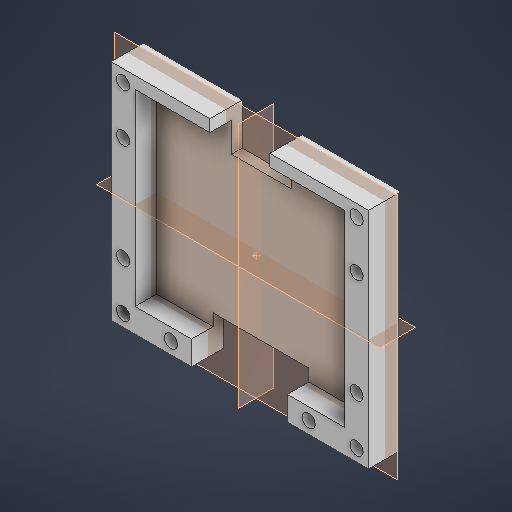
# Autodesk Inventor part: Checkpoint10.2_BackCover
Saved by Autodesk Inventor 2026.1 (Build 301233020, 233B)
## iProperties
Created: 2025-10-03
Part Number: Checkpoint10.2_BackCover
Material: Generic
Document SubType Name: Modeling
Designer: ghimirea
Density: 1 g/cm^3
Appearance: Default
Author: ghimirea
Autodesk Inventor part; units mm, degrees
sketch "Sketch1" plane through (0, 0, 0) normal (0, 0, 1) x (1, 0, 0)
  line L0 (-10.75, -9.35) -> (10.75, -9.35)
  line L1 (10.75, -9.35) -> (10.75, 9.35)
  line L2 (10.75, 9.35) -> (-10.75, 9.35)
  line L3 (-10.75, 9.35) -> (-10.75, -9.35)
  line L4 (-10.75, -9.35) -> (10.75, 9.35) construction
  line L5 (10.75, -9.35) -> (-10.75, 9.35) construction
  point P0 (0, 0)
  dimension "d0" = 21.5
  dimension "d1" = 18.7
  constraints: 12 end point, 2 midpoint, 2 parallel, 1 horizontal, 1 perpendicular
  measures "d0" distance of L0.start L0.end
  measures "d1" distance of L1.end L0.end
extrude "Extrusion1" add sketch "Sketch1" along normal mid plane 2.7
sketch "Sketch3" plane through (0, 0, 1.35) normal (0, 0, 1) x (1, 0, 0)
  line L0 (-8.75, -7.35) -> (8.75, -7.35)
  line L1 (8.75, -7.35) -> (8.75, 8.35)
  line L2 (8.75, 8.35) -> (-8.75, 8.35)
  line L3 (-8.75, 8.35) -> (-8.75, -7.35)
  line L4 (-8.75, -7.35) -> (8.75, 8.35) construction
  line L5 (8.75, -7.35) -> (-8.75, 8.35) construction
  line L6 (-10.75, -9.35) -> (10.75, -9.35)
  point P0 (0, 0.5)
  dimension "d8" = 17.5
  dimension "d47" = 2
  dimension "d61" = 15.7
  constraints: 14 end point, 2 midpoint
  measures "d8" distance of L0.start L0.end
  measures "d47" distance between parallel lines of L6 L0
  measures "d61" distance between parallel lines of L0 L2
extrude "Extrusion3" cut sketch "Sketch3" against normal blind 1.8
sketch "Sketch4" plane through (0, 0, 1.35) normal (0, 0, 1) x (1, 0, 0)
  line L0 (2.5, 5.884) -> (-2.5, 5.884)
  line L1 (-2.5, 5.884) -> (-2.5, 12.884)
  line L2 (-2.5, 12.884) -> (2.5, 12.884)
  line L3 (2.5, 12.884) -> (2.5, 5.884)
  line L4 (2.5, 5.884) -> (-2.5, 12.884) construction
  line L5 (-2.5, 5.884) -> (2.5, 12.884) construction
  point P0 (0, 0)
  point P1 (0, 9.384)
  dimension "d12" = 5
  dimension "d15" = 7
  constraints: 12 end point, 2 midpoint, 2 parallel, 1 horizontal, 1 perpendicular
  measures "d12" distance of L0.start L0.end
  measures "d15" distance between parallel lines of L0 L2
extrude "Extrusion4" cut sketch "Sketch4" against normal blind 3
sketch "Sketch7" plane through (-10.75, 0.5, 6.442) normal (1, 0, 0) x (0, -1, 0)
  line L0 (3.5, 6.442) -> (-2.5, 6.442)
  line L1 (-2.5, 6.442) -> (-2.5, 9.442)
  line L2 (-2.5, 9.442) -> (3.5, 9.442)
  line L3 (3.5, 9.442) -> (3.5, 6.442)
  line L4 (3.5, 6.442) -> (-2.5, 9.442) construction
  line L5 (-2.5, 6.442) -> (3.5, 9.442) construction
  line L6 (0.5, -1.8884) -> (0.5, 11.3304) projected
  line L7 (-8.85, 7.792) -> (-8.85, 5.092) projected
  point P0 (0, 0)
  point P1 (0.5, 7.942)
  point P2 (0.5, 7.942)
  point P3 (0.5, -1.8884)
  point P4 (0.5, 11.3304)
  point P5 (-8.85, 6.442)
  dimension "d24" = 6
  dimension "d23" = 3
  constraints: 12 end point, 4 midpoint, 2 parallel, 1 horizontal, 1 perpendicular, 1 point on line, 2 other
  measures "d24" distance of L0.start L0.end
  measures "d23" distance between parallel lines of L0 L2
extrude "Extrusion7" [suppressed]
fillet "Fillet1" [suppressed]
fillet "Fillet2" [suppressed]
fillet "Fillet3" [suppressed]
fillet "Fillet4" [suppressed]
fillet "Fillet5" [suppressed]
fillet "Fillet6" radius 0.2 1 edges at (10.75, 0, -1.35)
fillet "Fillet7" [suppressed]
fillet "Fillet8" [suppressed]
fillet "Fillet9" [suppressed]
fillet "Fillet10" [suppressed]
fillet "Fillet11" [suppressed]
mirror "Mirror2" [suppressed]
sketch "InsertPoles_Sketch" plane through (0, 0, 1.35) normal (0, 0, 1) x (1, 0, 0)
  circle A0 centre (-9.75, -8.35) radius 0.55
  line L0 (-10.75, 9.35) -> (-10.75, -9.35) projected
  line L1 (-10.75, -9.35) -> (10.75, -9.35) projected
  circle A1 centre (-9.75, -4.35) radius 0.55
  circle A2 centre (-9.75, 4.35) radius 0.55
  circle A3 centre (-9.75, 8.35) radius 0.55
  circle A4 centre (-5.75, -8.35) radius 0.55
  line L2 (-2.5, 9.35) -> (-10.75, 9.35) projected
  point P0 (0, 0)
  point P1 (-8.75, 9.35)
  dimension "d39" = 1.1
  dimension "d40" = 1
  dimension "d41" = 1
  dimension "d42" = 1.1
  dimension "d43" = 1.1
  dimension "d44" = 1.1
  dimension "d45" = 1.1
  dimension "d48" = 4
  dimension "d49" = 1
  dimension "d50" = 1
  dimension "d51" = 4
  dimension "d52" = 4
  constraints: 5 centre point
  measures "d39" diameter of A0
  measures "d40" distance from line of A0.centre L0
  measures "d41" distance from line of L1 A0.centre
  measures "d42" diameter of A1
  measures "d43" diameter of A2
  measures "d44" diameter of A3
  measures "d45" diameter of A4
  measures "d48" distance of A0.centre A1.centre
  measures "d49" distance from line of L2 A3.centre
  measures "d50" distance from line of L0 A3.centre
  measures "d51" distance of A2.centre A3.centre
  measures "d52" distance of A4.centre A0.centre
extrude "InsertPoles_Extrude" cut sketch "InsertPoles_Sketch" against normal blind 3
mirror "MirrorInsertPoles" about plane through (0, 0, 0) normal (1, 0, 0) of "InsertPoles_Extrude"
sketch "RibbonCableCutout_Sketch" plane through (0, 0, 1.35) normal (0, 0, 1) x (1, 0, 0)
  line L0 (3, -7.0087) -> (-3, -7.0087)
  line L1 (-3, -7.0087) -> (-3, -9.0087)
  line L2 (-3, -9.0087) -> (3, -9.0087)
  line L3 (3, -9.0087) -> (3, -7.0087)
  line L4 (3, -7.0087) -> (-3, -9.0087) construction
  line L5 (-3, -7.0087) -> (3, -9.0087) construction
  line L6 (0, 13.09) -> (0, -13.09) projected
  point P0 (0, 0)
  point P1 (0, -8.0087)
  point P2 (0, -8.0087)
  dimension "d56" = 6
  dimension "d57" = 2
  constraints: 12 end point, 3 midpoint, 2 parallel, 1 horizontal, 1 perpendicular, 1 point on line
  measures "d56" distance of L0.start L0.end
  measures "d57" distance of L1.end L0.end
extrude "RibbonCableCutout_Extrude" [suppressed]
fillet "Fillet12" [suppressed]
sketch "Sketch11" plane through (-0.0016, -9.35, -6.4418) normal (0, -1, 0) x (1, 0, 0)
  line L0 (3.9693, 3.0494) -> (-4.0307, 3.0494)
  line L1 (-4.0307, 3.0494) -> (-4.0307, 10.0494)
  line L2 (-4.0307, 10.0494) -> (3.9693, 10.0494)
  line L3 (3.9693, 10.0494) -> (3.9693, 3.0494)
  line L4 (3.9693, 3.0494) -> (-4.0307, 10.0494) construction
  line L5 (-4.0307, 3.0494) -> (3.9693, 10.0494) construction
  point P0 (0, 0)
  point P1 (-0.0307, 6.5494)
  dimension "d63" = 8
  dimension "d62" = 7
  constraints: 12 end point, 2 midpoint, 2 parallel, 1 horizontal, 1 perpendicular
  measures "d63" distance of L0.start L0.end
  measures "d62" distance between parallel lines of L0 L2
extrude "Extrusion10" cut sketch "Sketch11" against normal blind 3
